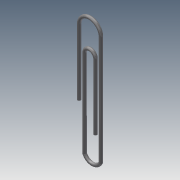
# Autodesk Inventor part: Paperclip
Saved by Autodesk Inventor 2015 (Build 190159000, 159)
## iProperties
Created: 2016-11-12
Part Number: Paperclip
Material: Aluminum 6061, Welded
Document SubType Name: Modeling
Designer: Aniket Pant
Density: 2.7 g/cm^3
Appearance: Stainless - Brushed
Author: Aniket Pant
Autodesk Inventor part; units mm, degrees
ref_plane "YZ Plane" through (0, 0, 0) normal (1, 0, 0) x (0, 1, 0)
ref_plane "XZ Plane" through (0, 0, 0) normal (0, 1, 0) x (-1, 0, 0)
sketch "Sketch1" plane through (0, 0, 0) normal (0, 0, 1) x (1, 0, 0)
  line L0 (0, 0) -> (0, 76.2)
  line L1 (25.4, 76.2) -> (25.4, -50.8)
  line L2 (6.35, -50.8) -> (6.35, 50.8)
  line L3 (19.05, 50.8) -> (19.05, -25.4)
  arc A0 (25.4, 76.2) -> (0, 76.2) centre (12.7, 76.2) ccw
  arc A1 (19.05, 50.8) -> (6.35, 50.8) centre (12.7, 50.8) ccw
  arc A2 (6.35, -50.8) -> (25.4, -50.8) centre (15.875, -46.835) ccw
  constraints: 8 end point, 6 point on circle, 4 tangent, 3 centre point, 1 parallel, 1 vertical
ref_plane "Work Plane1" through (0, 0, 0) normal (0, 1, 0) x (-1, 0, 0)
sketch "Sketch2" plane through (0, 0, 0) normal (0, 1, 0) x (-1, 0, 0)
  circle A0 centre (0, 0) radius 1.905
  dimension "d7" = 3.81
  constraints: 1 centre point, 1 coincident
  measures "d7" diameter of A0
sweep "Sweep1" add profiles "Sketch2" path "Sketch1"
body "Solid1"
